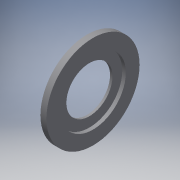
# Autodesk Inventor part: Washer
Saved by Autodesk Inventor 2019 Beta2 (Build 230110000, 110) ContinuousBuild 0
## iProperties
Created: 2012-08-08
Part Number: Washer
Material: Generic
Document SubType Name: Modeling
Designer: John
Density: 1 g/cm^3
Appearance: Default
Author: John
Autodesk Inventor part; units mm, degrees
ref_plane "YZ Plane" through (0, 0, 0) normal (1, 0, 0) x (0, 1, 0)
ref_plane "XZ Plane" through (0, 0, 0) normal (0, 1, 0) x (-1, 0, 0)
ref_plane "XY Plane" through (0, 0, 0) normal (0, 0, 1) x (1, 0, 0)
sketch "Sketch1" plane through (0, 0, 0) normal (1, 0, 0) x (0, 1, 0)
  circle A0 centre (0, 0) radius 4.953
  dimension "d0" = 9.906
  constraints: 1 centre point, 1 coincident
  measures "d0" diameter of A0
extrude "Extrusion1" add sketch "Sketch1" along normal blind 0.635
sketch "Sketch2" plane through (0.635, 0, 0) normal (1, 0, 0) x (0, 0, -1)
  circle A0 centre (0, 0) radius 4.953 projected
  circle A1 centre (0, 0) radius 3.4925
  dimension "d3" = 6.985
  constraints: 1 centre point, 1 coincident
  measures "d3" diameter of A1
extrude "Extrusion2" cut sketch "Sketch2" against normal blind 0.381 contours A1
sketch "Sketch3" plane through (0.254, 0, 0) normal (1, 0, 0) x (0, 0, -1)
  circle A0 centre (0, 0) radius 3.4925 projected
hole "Hole1" at (0.254, 0, 0) direction (-1, 0, 0) diameter 4.9022 end through all
body "Solid1"
